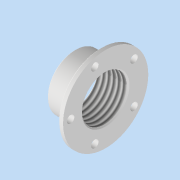
# Autodesk Inventor part: Gewinde Mutter Mitte
Saved by Autodesk Inventor 2021 (Build 250183000, 183)
## iProperties
Created: 2024-03-15
Part Number: Gewinde Mutter Mitte
Material: Generic
Document SubType Name: Modeling
Designer: Nokia
Density: 1 g/cm^3
Appearance: Default
Author: Nokia
Autodesk Inventor part; units mm, degrees
ref_plane "YZ Plane" through (0, 0, 0) normal (1, 0, 0) x (0, 1, 0)
ref_plane "XZ Plane" through (0, 0, 0) normal (0, 1, 0) x (-1, 0, 0)
ref_plane "XY Plane" through (0, 0, 0) normal (0, 0, 1) x (1, 0, 0)
sketch "Sketch1" plane through (0, 0, 0) normal (0, 0, 1) x (1, 0, 0)
  line L0 (0, 0) -> (0, 18)
  line L1 (0, 18) -> (-25, 18)
  line L2 (-25, 18) -> (-25, 22)
  line L3 (-25, 22) -> (-4, 22)
  line L4 (-4, 22) -> (-4, 34)
  line L5 (-4, 34) -> (0, 34)
  line L6 (0, 34) -> (0, 18)
  line L7 (0, 0) -> (-26.7257, 0)
  dimension "d0" = 18
  dimension "d1" = 25
  dimension "d2" = 4
  dimension "d3" = 21
  dimension "d4" = 12
  constraints: 16 end point, 5 perpendicular, 1 horizontal, 1 parallel, 1 point on line, 1 vertical
  measures "d0" distance of L0.start L0.end
  measures "d1" distance of L0.end L1.end
  measures "d2" distance of L1.end L2.end
  measures "d3" distance of L2.end L3.end
  measures "d4" distance of L3.end L4.end
revolve "Revolution1" add sketch "Sketch1" angle 360 about axis through (0, 0, 0) along (-1, 0, 0)
sketch "Sketch2" plane through (0, 0, 0) normal (1, 0, 0) x (0, 0, -1)
  circle A0 centre (0, 0) radius 34 projected
  line L0 (-34, 0) -> (-22, 0)
  circle A1 centre (0, 0) radius 22 projected
  circle A2 centre (-28, 0) radius 3
  circle A3 centre (-8.6525, -26.6296) radius 3
  circle A4 centre (22.6525, -16.458) radius 3
  circle A5 centre (22.6525, 16.458) radius 3
  circle A6 centre (-8.6525, 26.6296) radius 3
  dimension "d6" = 6
  dimension "d9" = 360
  constraints: 5 centre point, 2 end point, 2 horizontal alignment, 1 horizontal, 1 midpoint, 13 other
  measures "d6" diameter of A2
hole "Hole1" at (0, 0, 28) at (0, 26.6296, 8.6525) at (0, 16.458, -22.6525) at (0, -16.458, -22.6525) at (0, -26.6296, 8.6525) direction (-1, 0, 0) diameter 6 end through all
thread "Thread1" size "M36x4" class "6H" standard "ANSI Metric M Profile" length 50
chamfer "Chamfer1" distance 1 angle 45 4 edges at (0, -18, 0) (-25, -18, 0) (-25, -22, 0) (-4, -34, 0)
body "Solid1"
